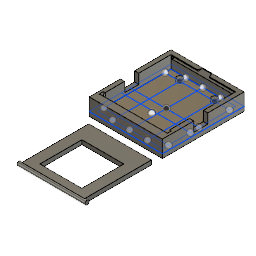
Parametric Sensor Box with Lid v0.0.18 (For Sparkfun Spectral Triad large window example) (Autodesk Fusion 360 design; units mm, degrees)
Autodesk Fusion 360 part; units mm, degrees
sketch "Spectral Triad Sensor Box" plane through (0, 0, 0) normal (0, 1, 0) x (1, 0, 0) in component "Spectral Triad Sensor Box v0.0.18"
  line L0 (-19.7961, -0.0903) -> (17.2039, -0.0903)
  line L1 (17.2039, -0.0903) -> (17.2039, 41.9097)
  line L2 (17.2039, 41.9097) -> (-19.7961, 41.9097)
  line L3 (-19.7961, 41.9097) -> (-19.7961, -0.0903)
  line L4 (-22.2961, 44.4097) -> (-22.2961, -2.5903)
  line L5 (-22.2961, -2.5903) -> (19.7039, -2.5903)
  line L6 (19.7039, -2.5903) -> (19.7039, 44.4097)
  line L7 (19.7039, 44.4097) -> (-22.2961, 44.4097)
  line L8 (8.7039, -0.0903) -> (8.7039, 41.9097)
  line L9 (-11.2961, 41.9097) -> (-11.2961, -0.0903)
  line L10 (-19.7961, 3.4097) -> (17.2039, 3.4097)
  line L11 (17.2039, 38.4097) -> (-19.7961, 38.4097)
  line L12 (-1.5461, 41.9097) -> (-1.5461, -0.0903)
  line L13 (-19.7961, 20.9097) -> (17.2039, 20.9097)
  circle A0 centre (-11.2961, 38.4097) radius 1.6
  circle A1 centre (8.7039, 38.4097) radius 1.6
  line L14 (17.2039, 15.9097) -> (-19.7961, 15.9097)
  line L15 (-19.7961, 20.9097) -> (-22.2961, 20.9097)
  line L16 (-22.2961, 20.9097) -> (19.7039, 20.9097)
  line L17 (-19.7961, 15.9097) -> (-22.2961, 15.9097)
  line L18 (-22.2961, 15.9097) -> (19.7039, 15.9097)
  point P0 (-1.5461, 20.9097)
  point P1 (-3.4221, 14.4673)
  dimension "d82" = 37
  dimension "d83" = 42
  dimension "d84" = 2.5
  dimension "d99" = -18.25
  dimension "d100" = -21
  dimension "d101" = 3.2
  dimension "d102" = 3.2
  dimension "d204" = 2.5
  constraint horizontal L0
  constraint vertical L1
  constraint horizontal L2
  constraint vertical L3
  constraint coincident L12 P0
  constraint coincident L13 P0
  constraint coincident L9 A0.centre
  constraint coincident L11 A0.centre
  constraint coincident L8 A1.centre
  constraint coincident L11 A1.centre
  constraint perpendicular L4 L15
  constraint midpoint L6 L16.end
  constraint coincident L4 L17.end
  constraint perpendicular L4 L17
  constraint coincident L6 L18.end
  constraint perpendicular L6 L18
  measures "d82" distance of L0.start L0.end
  measures "d83" distance of L0.start L2.end
  measures "d101" diameter of A0
  measures "d102" diameter of A1
  measures "d204" distance of L13.start L15.end
extrude "Extrude16" add sketch "Spectral Triad Sensor Box" along normal blind 1.65 contours L9 L11 A0 | L9 L11 A0 | L9 L11 A0 | L9 L11 A0 | L8 L11 A1 | L8 L11 A1 | L8 L11 A1 | L8 L11 A1 makes body 1 at (-10.0704, 1.1, -39.4382) makes body 2 at (7.4285, 1.1, -39.3758) in component "Spectral Triad Sensor Box v0.0.18"
extrude "Extrude3" add sketch "Spectral Triad Sensor Box" against normal blind 2.5 separate body makes body 3 in component "Spectral Triad Sensor Box v0.0.18"
extrude "Extrude2" add sketch "Spectral Triad Sensor Box" along normal blind 7.25 separate body contours L0 L1 L3 L4 L5 L6 L17 L18 | L3 L4 L15 L16 L17 L18 | L1 L2 L3 L4 L6 L7 L15 L16 | L1 L6 L16 L18 makes body 4 in component "Spectral Triad Sensor Box v0.0.18"
sketch "Sketch1" plane through (0, 0, 0) normal (0, 1, 0) x (1, 0, 0)
sketch "Sketch2" plane through (0, 0, 0) normal (0, 1, 0) x (1, 0, 0)
sketch "Sketch2 (2)" plane through (0, 0, 0.0903) normal (0, 0, -1) x (-1, 0, 0) in component "Spectral Triad Sensor Box v0.0.18"
  line L0 (-17.2039, 0) -> (19.7961, 0)
  line L1 (19.7961, 7.25) -> (-17.2039, 7.25)
  line L2 (-17.2039, 2.15) -> (19.7961, 2.15)
  line L3 (19.7961, 0) -> (19.7961, 7.25)
  line L4 (-17.2039, 7.25) -> (-17.2039, 0)
  dimension "d103" = -2.15
extrude "Extrude4" add sketch "Sketch2 (2)" along normal blind 3 contours L1 L2 L3 L4 bodies 4 in component "Spectral Triad Sensor Box v0.0.18"
chamfer "Chamfer1" distance 2.5 angle 45 1 edges at (-1.2961, 2.15, -2.9097) on bodies 4 in component "Spectral Triad Sensor Box v0.0.18"
ref_plane "WorkPlane1" through (-1.2961, 4.65, -2.9097) normal (0, -1, 0) x (1, 0, 0) in component "Spectral Triad Sensor Box v0.0.18"
sketch "Sketch3" plane through (-1.1524, 4.65, -12.0435) normal (0, -1, 0) x (1, 0, 0) in component "Spectral Triad Sensor Box v0.0.18"
combine "Combine1" operation add target body 3 tool bodies 4 keep tools in component "Spectral Triad Sensor Box v0.0.18"
sketch "Sketch3 (2)" plane through (0, 0, -41.9097) normal (0, 0, 1) x (1, 0, 0)
  line L0 (-19.7961, 0) -> (17.2039, 0)
  line L1 (17.2039, 0) -> (17.2039, 7.25)
  line L2 (17.2039, 7.25) -> (-19.7961, 7.25)
  line L3 (-19.7961, 7.25) -> (-19.7961, 0)
  line L4 (17.2039, 6.8333) -> (-19.7961, 6.8333)
  line L5 (-19.7961, 6.8333) -> (12.2036, 6.8333)
  line L6 (12.2036, 6.8333) -> (12.2036, 5.5)
  line L7 (12.2036, 5.5) -> (-19.7961, 5.5)
  line L8 (-19.7961, 5.5) -> (-19.7961, 6.8333)
  dimension "d110" = -0.4167
  dimension "d111" = 1.3333
  constraint horizontal L5
  constraint vertical L6
  constraint horizontal L7
  constraint vertical L8
  measures "d111" distance of L4.end L7.end
extrude "Extrude5" add sketch "Sketch3 (2)" along normal blind 1.6667 draft -45 contours L3 L4 L5 L6 L7 L8 bodies 3 4 in component "Spectral Triad Sensor Box v0.0.18"
delete_face "DeleteFace1" 4 faces at (11.9814, 6.1667, -41.6875) (-8.9073, 6.6111, -41.6875) (1.3148, 5.7222, -41.6875) (-19.5738, 6.1667, -41.6875) on bodies 3 in component "Spectral Triad Sensor Box v0.0.18"
sketch "Sketch4" plane through (0, 0, -41.9097) normal (0, 0, 1) x (1, 0, 0) in component "Spectral Triad Sensor Box v0.0.18"
  line L0 (-19.7961, 7.25) -> (-19.7961, 0)
  line L1 (-19.7961, 0) -> (17.2039, 0)
  line L2 (17.2039, 0) -> (17.2039, 7.25)
  line L3 (17.2039, 7.25) -> (-19.7961, 7.25)
  line L4 (17.2039, 4.75) -> (-19.7961, 4.75)
  line L5 (-19.7961, 4.75) -> (17.2039, 4.75)
  line L6 (-19.7961, 4.75) -> (17.2039, 4.75) construction
  line L7 (17.2039, 7.25) -> (-19.7961, 7.25) construction
  line L8 (16.7039, 0) -> (16.7039, 6.75) construction
  line L9 (16.7039, 6.75) -> (-19.2961, 6.75) construction
  line L10 (-19.2961, 6.75) -> (-19.2961, 0) construction
  line L11 (17.2039, 5.25) -> (-19.7961, 5.25) construction
  line L12 (-19.2961, 6.75) -> (16.7039, 6.75) construction
  line L13 (16.7039, 6.75) -> (16.7039, 5.25) construction
  line L14 (16.7039, 5.25) -> (-19.2961, 5.25) construction
  line L15 (-19.2961, 5.25) -> (-19.2961, 6.75) construction
  line L16 (-19.2961, 6.75) -> (16.7039, 6.75)
  line L17 (16.7039, 6.75) -> (16.7039, 5.25)
  line L18 (16.7039, 5.25) -> (-19.2961, 5.25)
  line L19 (-19.2961, 5.25) -> (-19.2961, 6.75)
  line L20 (-1.2961, 7.25) -> (-1.2961, 0)
  circle A0 through (2.4539, 5.25, 0) (-3.1711, 7.5464, -2.2964) (-3.1711, 2.9536, 2.2964)
  dimension "d198" = -18.5
  constraint coincident L2.end L3.start
  constraint coincident L0.start L3.end
  constraint horizontal L12
  constraint vertical L13
  constraint horizontal L14
  constraint vertical L15
  constraint coincident L8 L13.end
  constraint coincident L11 L13.end
  constraint horizontal L16
  constraint vertical L17
  constraint horizontal L18
  constraint vertical L19
extrude "Extrude14" cut sketch "Sketch4" along normal blind 5 contours L18 A0 | L18 A0 in plane through (0, 2.625, -39.2847) normal (0, 0.707107, 0.707107) bodies 3 in component "Spectral Triad Sensor Box v0.0.18"
ref_plane "WorkPlane2" through (-1.2961, 3.625, -20.9097) normal (1, 0, 0) x (0, 0, -1) in component "Spectral Triad Sensor Box v0.0.18"
sketch "Sketch1 (2)" plane through (0, 0, 0) normal (0, 1, 0) x (1, 0, 0) in component "Spectral Triad Sensor Box Lid v0.0.18"
  line L0 (-13.6773, 0.3047) -> (24.8227, 0.3047)
  line L1 (24.8227, 0.3047) -> (24.8227, -35.6953)
  line L2 (24.8227, -35.6953) -> (-13.6773, -35.6953)
  line L3 (-13.6773, -35.6953) -> (-13.6773, 0.3047)
  dimension "d118" = 38.5
  dimension "d119" = 36
  constraint horizontal L0
  constraint vertical L1
  constraint horizontal L2
  constraint vertical L3
  measures "d118" distance of L0.start L0.end
  measures "d119" distance of L0.start L2.end
extrude "Extrude1" add sketch "Sketch1 (2)" along normal blind 2.5 separate body makes body 5 in component "Spectral Triad Sensor Box Lid v0.0.18"
sketch "Sketch2 (3)" plane through (24.8227, 0, 0) normal (1, 0, 0) x (0, 0, -1) in component "Spectral Triad Sensor Box Lid v0.0.18"
sketch "Sketch6" plane through (0, 0, -2.9097) normal (0, 0, -1) x (-1, 0, 0) in component "Spectral Triad Sensor Box v0.0.18"
  line L0 (-17.2039, 4.65) -> (19.7961, 4.65)
  line L1 (19.7961, 4.65) -> (19.7961, 7.25)
  line L2 (19.7961, 7.25) -> (-17.2039, 7.25)
  line L3 (-17.2039, 7.25) -> (-17.2039, 4.65)
  line L4 (19.7961, 6.25) -> (-17.2039, 6.25)
  circle A0 through (-17.2039, 6.25, -1.5) (-17.2039, 7.549, 0.75) (-17.2039, 4.951, 0.75)
extrude "Extrude11" cut sketch "Sketch6" against normal blind 1 contours A0 in plane through (17.2039, 0, -2.9097) normal (-1, 0, 0) bodies 3 in component "Spectral Triad Sensor Box v0.0.18"
extrude "Extrude10" cut sketch "Sketch4" against normal blind 1.25 draft -45 contours L16 L18 L19 L20 | L16 L17 L18 L20 bodies 3 in component "Spectral Triad Sensor Box v0.0.18"
move_body "Move1" bodies 5 to x (1, 0, 0) y (0, 1, 0) z (0, 0, 1) at (-6.8059, 0, 10.504) in component "Spectral Triad Sensor Box Lid v0.0.18"
extrude "Extrude12" cut 1 faces at (18.2039, 5.4767, -3.0779) along direction (-1, 0, 0) blind 39 on bodies 3 bodies 3 in component "Spectral Triad Sensor Box v0.0.18"
sketch "Sketch4 (2)" plane through (0, 0, 35.8782) normal (0, 0, -1) x (-1, 0, 0)
  line L0 (18.7961, -3) -> (18.7961, -0.5)
  line L1 (18.7961, -0.5) -> (-17.2039, -0.5)
  line L2 (-17.2039, -0.5) -> (-17.2039, -3)
  line L3 (-17.2039, -3) -> (18.7961, -3)
  line L4 (18.2961, -2.5) -> (18.2961, -1)
  line L5 (18.2961, -1) -> (-16.7039, -1)
  line L6 (-16.7039, -1) -> (-16.7039, -2.5)
  line L7 (-16.7039, -2.5) -> (18.2961, -2.5)
extrude "Extrude8" add sketch "Sketch4 (2)" along normal blind 1.25 draft -45 contours L4 L5 L6 L7 sketch seen with x (0, 0, -1) y (0, 1, 0) z (1, 0, 0) at (-56.3614, 3, 27.4032) bodies 5 in component "Spectral Triad Sensor Box Lid v0.0.18"
sketch "Sketch5" plane through (17.2039, 0, 0) normal (1, 0, 0) x (0, 0, -1)
  line L0 (-74.3782, -3) -> (-35.8782, -3)
  line L1 (-35.8782, -3) -> (-35.8782, -0.5)
  line L2 (-35.8782, -0.5) -> (-74.3782, -0.5)
  line L3 (-74.3782, -0.5) -> (-74.3782, -3)
  line L4 (-35.8782, -1.75) -> (-74.3782, -1.75)
  circle A0 centre (-74.3782, -1.75) radius 1.5
  dimension "d173" = -1.25
  dimension "d174" = 3
  constraint coincident L4.end A0.centre
  measures "d174" diameter of A0
sketch "Sketch6 (2)" plane through (30.4032, -3, 81.1841) normal (0, 0, 1) x (0, 1, 0)
sketch "Sketch7" plane through (0, -0.5, 0) normal (0, 1, 0) x (-1, 0, 0)
  line L0 (15.7961, 35.8782) -> (15.7961, 74.3782)
  line L1 (-20.2039, 74.3782) -> (-20.2039, 35.8782)
  line L2 (-20.2039, 35.8782) -> (15.7961, 35.8782)
  line L3 (-14.2039, 74.3782) -> (-14.2039, 35.8782)
  line L4 (15.7961, 67.299) -> (-20.2039, 67.299)
  line L5 (-14.2039, 67.299) -> (9.7961, 67.299)
  line L6 (9.7961, 67.299) -> (9.7961, 43.299)
  line L7 (9.7961, 43.299) -> (-14.2039, 43.299)
  line L8 (-14.2039, 43.299) -> (-14.2039, 67.299)
  line L9 (15.7961, 74.3782) -> (-20.2039, 74.3782)
  dimension "d181" = 24
  dimension "d182" = 24
  constraint horizontal L5
  constraint vertical L6
  constraint horizontal L7
  constraint vertical L8
  constraint coincident L3 L5.start
  constraint coincident L4 L5.start
  measures "d181" distance of L5.start L5.end
  measures "d182" distance of L5.start L7.end
sketch "Sketch4 (3)" plane through (18.0168, 0, 0) normal (1, 0, 0) x (0, 0, -1) in component "Spectral Triad Sensor Box Lid v0.0.18"
  line L0 (-46.1993, 0) -> (-10.1993, 0)
  line L1 (-10.1993, 0) -> (-10.1993, 2.5)
  line L2 (-10.1993, 2.5) -> (-46.1993, 2.5)
  line L3 (-46.1993, 2.5) -> (-46.1993, 0)
  line L4 (-10.1993, 1.25) -> (-46.1993, 1.25)
  circle A0 through (-46.1993, 1.25, -1.25) (-46.1993, 2.3325, 0.625) (-46.1993, 0.1675, 0.625)
extrude "Extrude12'" add sketch "Sketch4 (3)" against normal blind 1.5 contours L3 A0 | L3 A0 in plane through (18.0168, 0, 46.1993) normal (0, 0, -1) bodies 5 in component "Spectral Triad Sensor Box Lid v0.0.18"
extrude "Extrude13" add 1 faces at (18.3002, 1.5554, 47.6993) along direction (0, 0, -1) blind 39 on bodies 5 bodies 5 in component "Spectral Triad Sensor Box Lid v0.0.18"
sketch "Sketch5 (2)" plane through (0, 2.5, 0) normal (0, 1, 0) x (-1, 0, 0) in component "Spectral Triad Sensor Box Lid v0.0.18"
  line L0 (20.4832, 46.1993) -> (-18.0168, 46.1993)
  line L1 (-18.0168, 46.1993) -> (-18.0168, 10.1993)
  line L2 (-18.0168, 10.1993) -> (20.4832, 10.1993)
  line L3 (20.4832, 10.1993) -> (20.4832, 46.1993)
  line L4 (10.4832, 10.1993) -> (10.4832, 46.1993)
  line L5 (20.4832, 40.1993) -> (-18.0168, 40.1993)
  line L6 (10.4832, 40.1993) -> (-13.5168, 40.1993)
  line L7 (-13.5168, 40.1993) -> (-13.5168, 16.1993)
  line L8 (-13.5168, 16.1993) -> (10.4832, 16.1993)
  line L9 (10.4832, 16.1993) -> (10.4832, 40.1993)
  dimension "d194" = 24
  dimension "d195" = 24
  constraint horizontal L6
  constraint vertical L7
  constraint horizontal L8
  constraint vertical L9
  constraint coincident L4 L6.start
  constraint coincident L5 L6.start
  measures "d194" distance of L6.start L6.end
  measures "d195" distance of L6.start L8.end
extrude "Extrude14'" cut sketch "Sketch5 (2)" against normal blind 2.5 contours L4 L5 L6 L7 L8 L9 bodies 5 in component "Spectral Triad Sensor Box Lid v0.0.18"
sketch "Sketch3 (3)" plane through (0, 7.25, 0) normal (0, 1, 0) x (-1, 0, 0) in component "Spectral Triad Cowl Component"
  line L0 (-18.2039, -1.7917) -> (20.7961, -1.7917)
  line L1 (19.7961, -4.0278) -> (19.7961, -41.9097)
  line L2 (19.7961, -41.9097) -> (4.7692, -41.9097)
  line L3 (-17.2039, -41.9097) -> (-17.2039, -4.0278)
  line L4 (-18.2039, -4.0278) -> (-18.2039, -1.7917)
  line L5 (-19.7039, -44.4097) -> (22.2961, -44.4097)
  line L6 (22.2961, -44.4097) -> (22.2961, 2.5903)
  line L7 (22.2961, 2.5903) -> (-19.7039, 2.5903)
  line L8 (-19.7039, 2.5903) -> (-19.7039, -44.4097)
  line L9 (-19.7039, -23.4097) -> (22.2961, -23.4097)
  line L10 (-19.7039, -15.4097) -> (22.2961, -15.4097)
  ellipse E0 centre (1.2961, -39.9097) end of major axis (1.2961, -45.213) minor radius 3.75 (3.7583, -43.9097) -> (4.7692, -41.9097) ccw construction
  line L11 (3.7583, -43.9097) -> (-1.1661, -43.9097)
  ellipse E1 centre (1.2961, -39.9097) end of major axis (1.2961, -45.213) minor radius 3.75 (-2.177, -41.9097) -> (-1.1661, -43.9097) ccw construction
  line L12 (-2.177, -41.9097) -> (-17.2039, -41.9097)
  line L13 (-17.2039, -4.0278) -> (-18.2039, -4.0278)
  line L14 (20.7961, -1.7917) -> (20.7961, -4.0278)
  line L15 (20.7961, -4.0278) -> (19.7961, -4.0278)
extrude "Extrude15" cut sketch "Sketch3 (3)" against normal blind 5.6 contours L3 L8 L9 L10 | L1 L6 L9 L10 bodies 3 in component "Spectral Triad Sensor Box v0.0.18"
move_body "Move2" bodies 5 to x (1, 0, 0) y (0, 1, 0) z (0, 0, 1) at (-27.1469, 0, 4.8755) in component "Spectral Triad Sensor Box Lid v0.0.18"
component "Spectral Triad Cowl Component" placed x (1, 0, 0) y (0, 1, 0) z (0, 0, 1) at (0, 0, 0)
component "Spectral Triad Sensor Box v0.0.18" placed x (1, 0, 0) y (0, 1, 0) z (0, 0, 1) at (0, 0, 0) in component "Spectral Triad Cowl Component"
component "Spectral Triad Sensor Box Lid v0.0.18" placed x (0, 0, 1) y (0, 1, 0) z (-1, 0, 0) at (30.4032, -3, 56.3614) in component "Spectral Triad Sensor Box v0.0.18"
equation "PCBWidth = 36 mm" comment "Total width of PCB."
equation "PCBHeight = 41 mm" comment "Total height (external) of PCB."
equation "PCBThick = 1.65 mm" comment "Thicknes (or depth) of the PCB. Just the PCB--Nothing else. Most PCBs are 1.65 mm. (But I know some substrates vary.)"
equation "PCBMaxThick = 4.75 mm" comment "Thickness of board plus any connectors (e.g. Qwiic in original project). This should *include* the PCBThick above, so will always be greater."
equation "PCBMountHoleVOffset = 3 mm" comment "Vertical Offset from top edge of PCB to center of mounting hole. Used to create the posts that allow PCB to \"snap in\"."
equation "PCBMountHoleDiameter = 3.2 mm" comment "Diameter of holes that screws normally go in."
equation "Shell = 2.5 mm" comment "Thickness of the shell/walls for lid and box."
equation "Gap = 0.5 mm" comment "Gap between fitting parts. Increase for lower-quality printer. Decrease for super-tight fit. (Must be positive!) Also used to calculate hinge pin/receptacle size, so change with care."
equation "SidePlugWidth = 8 mm" comment "Exact width of the adapter/connection/cable, etc. I recommend the larger of connector or cable width. 0 = none."
equation "SidePlugOffset = 18 mm" comment "Offset from the top of board for plugs/cables, etc. Currently must be on both sides. (If you're reading this, I like to add about \"Gap * 2\" here, because we want the gap on both sides of the connector/adapter plug(s). 0 = very \"top\" of lid (opposite hinge)."
equation "PCBMountHoleHOffset = 8 mm" comment "Horizontal Offset from left & right edges of PCB to center of mounting hole."
equation "d82 = PCBWidth + ( Gap * 2 )"
equation "d83 = PCBHeight + ( Gap * 2 )"
equation "d84 = Shell"
equation "d85 = -( PCBMountHoleHOffset + Gap )"
equation "d86 = -( PCBMountHoleHOffset + Gap )"
equation "d87 = -( PCBMountHoleVOffset + Gap )"
equation "d88 = -( PCBMountHoleVOffset + Gap )"
equation "d95 = PCBMaxThick + Shell"
equation "d97 = -Shell"
equation "d99 = -( PCBWidth + Gap ) / 2"
equation "d100 = -( PCBHeight + ( Gap * 2 ) ) / 2"
equation "d101 = PCBMountHoleDiameter"
equation "d102 = PCBMountHoleDiameter"
equation "d103 = -( PCBThick + 0.5 mm )"
equation "BoardOverhang = 3 mm" comment "Total size of overhang at widest part. (Amount that \"grips\" the board will always be calculated at 0.5, for now.)"
equation "d105 = BoardOverhang"
equation "d107 = ( BoardOverhang - 0.5 mm )"
equation "d110 = -( Shell / 6 )"
equation "d112 = ( Shell / 3 ) * 2"
equation "d118 = PCBHeight - BoardOverhang + Gap"
equation "d119 = PCBWidth"
equation "d120 = Shell"
equation "LidWindowHSize = 24 mm" comment "Width of window in the lid. 0 = none."
equation "LidWindowVSize = 24 mm" comment "Height of window in lid. 0 = none."
equation "LidWindowHOffset = 6 mm" comment "Offset from left edge of lid to left side of window. 0 = place at very left edge."
equation "LidWindowVOffset = 10 mm" comment "Offset from top edge of lid to top side of window. 0 = place at very top of lid."
equation "d153 = LidWindowHSize"
equation "d156 = -Shell"
equation "d157 = -Gap"
equation "d158 = -( Shell - Gap )"
equation "d159 = -( Shell / 2 )"
equation "d165 = Gap * 2"
equation "d167 = PCBWidth + ( Gap * 6 )"
equation "d170 = -Gap"
equation "d171 = Shell / 2"
equation "d173 = -Shell / 2"
equation "d179 = -LidWindowHOffset"
equation "d181 = LidWindowVSize"
equation "d182 = LidWindowHSize"
equation "d187 = -( Gap * 3 )"
equation "d189 = -( PCBWidth + ( Gap * 6 ) )"
equation "d191 = -( SidePlugOffset + SidePlugWidth )"
equation "d192 = -LidWindowVOffset"
equation "d193 = -LidWindowHOffset"
equation "d194 = LidWindowVSize"
equation "d195 = LidWindowHSize"
equation "d196 = -Shell"
equation "d198 = -( PCBWidth / 2 + Gap )"
equation "d202 = Shell * 2"
equation "d205 = -( Shell + Gap + SidePlugOffset )"
equation "d206 = -( Shell + Gap + SidePlugOffset + SidePlugWidth )"
equation "d207 = -( PCBMaxThick - PCBThick + Shell )"
equation "d209 = PCBThick"
